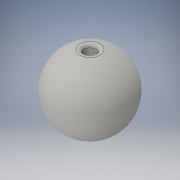
# Autodesk Inventor part: float
Saved by Autodesk Inventor 2016 SP1 (Build 200210100, 210)
## iProperties
Created: 2015-12-07
Part Number: float
Material: Generic
Document SubType Name: Modeling
Designer: steele
Density: 1 g/cm^3
Appearance: Default
Author: steele
Autodesk Inventor part; units mm, degrees
ref_plane "YZ Plane" through (0, 0, 0) normal (1, 0, 0) x (0, 1, 0)
ref_plane "XZ Plane" through (0, 0, 0) normal (0, 1, 0) x (-1, 0, 0)
ref_plane "XY Plane" through (0, 0, 0) normal (0, 0, 1) x (1, 0, 0)
sketch "Sketch8" plane through (0, 0, 0) normal (0, 0, 1) x (1, 0, 0)
  arc A0 (0, -38.1) -> (0, 38.1) centre (0, 0) ccw
  line L0 (0, 38.1) -> (0, -38.1)
  line L1 (0, -53.34) -> (0, 53.34) projected
  dimension "d25" = 76.2
  constraints: 2 end point, 2 point on circle, 1 centre point, 1 coincident
  measures "d25" diameter of A0
revolve "Revolution1" add sketch "Sketch8" angle 360 about axis through (0, -10, 0) along (0, 1, 0)
sketch "Sketch9" plane through (0, 0, 0) normal (0, 1, 0) x (-1, 0, 0)
  circle A0 centre (0, 0) radius 6.35
  dimension "d27" = 12.7
  constraints: 1 centre point, 1 coincident
  measures "d27" diameter of A0
extrude "Extrusion4" cut sketch "Sketch9" along normal mid plane 76.2
fillet "Fillet1" radius 3.175 4 edges at (0, 37.5671, 6.35) (0, 37.5671, -6.35) (0, -37.5671, -6.35) (0, -37.5671, 6.35)
equation "\"d25\" = ballDiam"
equation "\"d27\" = holeDiam"
equation "\"d28\" = ballDiam"
equation "\"ballDiam\" = 76.2"
equation "\"holeDiam\" = 12.7"
body "Solid3"
